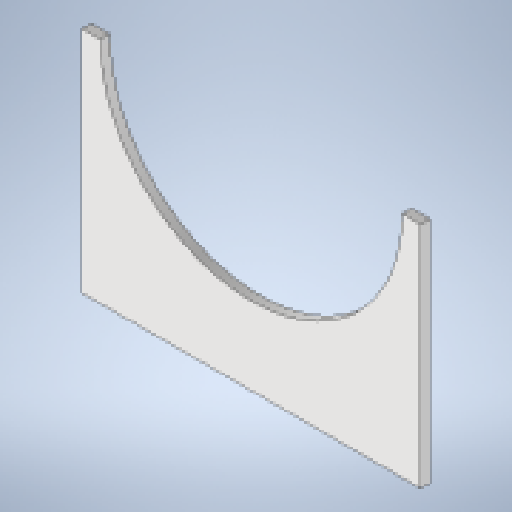
# Autodesk Inventor part: ДМФ 091 Постель НОС v2.0
Saved by Autodesk Inventor 2025 (Build 290162010, 162A)
## iProperties
Created: 2024-04-28
Part Number: ДМФ 091 Постель НОС v2.0
Material: Generic
Document SubType Name: Sheet Metal
Designer: admin
Density: 1 g/cm^3
Appearance: Default
Stock Number: Постель_Нос
Sheet Metal Rule: Default
Sheet Metal Width: 0,000 mm
Sheet Metal Length: 0,000 mm
Sheet Metal Area: 0,000 mm^2
Author: pokla
Autodesk Inventor part; units mm, degrees
ref_plane "YZ Plane" through (0, 0, 0) normal (1, 0, 0) x (0, 1, 0)
ref_plane "XZ Plane" through (0, 0, 0) normal (0, 1, 0) x (-1, 0, 0)
ref_plane "XY Plane" through (0, 0, 0) normal (0, 0, 1) x (1, 0, 0)
sketch "Sketch1" plane through (0, 0, 0) normal (0, 0, 1) x (1, 0, 0)
  line L0 (0, 211.738) -> (0, 171) construction
  line L1 (0, 211.738) -> (0, 171) construction
  circle A0 centre (0, 0) radius 171
  line L2 (-171, 0) -> (-191, 0)
  line L3 (-191, 0) -> (-191, -250)
  line L4 (-191, -250) -> (191, -250)
  line L5 (191, -250) -> (191, 0)
  line L6 (191, 0) -> (171, 0)
  dimension "d46" = 342
  dimension "d47" = 20
  dimension "d49" = 250
  measures "d46" diameter of A0
  measures "d47" distance of L2.start L2.end
  measures "d49" distance of L4.end L5.end
extrude "Plate1" add sketch "Sketch1" along normal blind 10 contours L6 L5 L4 L3 L2 A0
equation "\"d50\" = Thickness"
equation "\"BendReliefDepth\" = 0.5 * Thickness"
equation "\"Thickness\" = 10"
body "Solid2"
